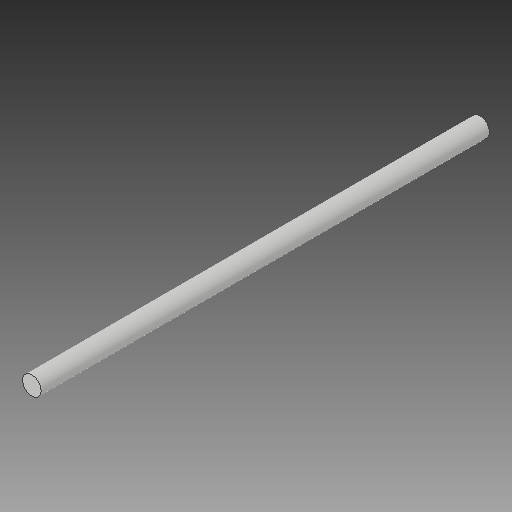
# Autodesk Inventor part: turntable_retention_shaft
Saved by Autodesk Inventor 2019 (Build 230136000, 136)
## iProperties
Created: 2019-05-16
Part Number: turntable_retention_shaft
Material: Generic
Document SubType Name: Modeling
Designer: Nathan
Density: 1 g/cm^3
Appearance: Default
Author: Nathan
Autodesk Inventor part; units mm, degrees
ref_plane "YZ Plane" through (0, 0, 0) normal (1, 0, 0) x (0, 1, 0)
ref_plane "XZ Plane" through (0, 0, 0) normal (0, 1, 0) x (-1, 0, 0)
ref_plane "XY Plane" through (0, 0, 0) normal (0, 0, 1) x (1, 0, 0)
sketch "Sketch1" plane through (0, 0, 0) normal (0, 0, 1) x (1, 0, 0)
  circle A0 centre (0, 0) radius 3.175
  dimension "d0" = 6.35
  constraints: 1 centre point, 1 coincident
  measures "d0" diameter of A0
extrude "Extrusion1" add sketch "Sketch1" along normal blind 152.4
equation "\"d0\" = turntable_retention_shaft_diameter"
equation "\"d1\" = turntable_retention_shaft_length"
equation "\"base_length\" = 177.8"
equation "\"base_width\" = 127"
equation "\"base_height\" = 12.7"
equation "\"base_cutout_contact_angle\" = 70deg"
equation "\"base_cutout_diameter\" = 44.45"
equation "\"turntable_motor_support_thickness\" = 3.175"
equation "\"turntable_motor_support_width\" = 63.5"
equation "\"turntable_motor_support_height\" = 19.05"
equation "\"turntable_motor_boss\" = 25.4"
equation "\"turntable_bed_depth\" = 3.175"
equation "\"turntable_diameter\" = 101.6"
equation "\"turntable_height\" = 9.525"
equation "\"turntable_spur_width\" = 6.35"
equation "\"turntable_retention_shaft_diameter\" = 6.35"
equation "\"spine_diameter\" = 31.75"
equation "\"spine_height\" = 25.4"
equation "\"shoulder_length\" = 50.8"
equation "\"shoulder_width\" = 69.85"
equation "\"shoulder_wall_thickness\" = 4.7625"
equation "\"shoulder_gear_diameter\" = 63.5"
equation "\"shoulder_motor_gear_diameter\" = 25.4"
equation "\"shoulder_gear_shaft_diameter\" = 12.7"
equation "\"shoulder_motor_boss\" = 25.4"
equation "\"turntable_retention_shaft_length\" = 152.4"
equation "\"arm_distal_length\" = 152.4"
equation "\"arm_proximal_central_diameter\" = 25.4"
equation "\"arm_proximal_length\" = 203.2"
equation "\"shoulder_gear_thickness\" = 6.35"
equation "\"arm_proximal_thickness\" = 9.525"
equation "\"arm_proximal_motor_boss\" = 25.4"
body "Solid1"
